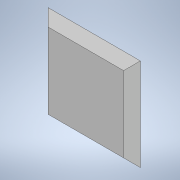
# Autodesk Inventor part: clear-square
Saved by Autodesk Inventor 2021 (Build 250183000, 183)
## iProperties
Created: 2020-12-08
Part Number: clear-square
Material: Generic
Document SubType Name: Modeling
Designer: Luke Kamols
Density: 1 g/cm^3
Appearance: Default
Author: Luke Kamols
Autodesk Inventor part; units mm, degrees
ref_plane "YZ Plane" through (0, 0, 0) normal (1, 0, 0) x (0, 1, 0)
ref_plane "XZ Plane" through (0, 0, 0) normal (0, 1, 0) x (-1, 0, 0)
ref_plane "XY Plane" through (0, 0, 0) normal (0, 0, 1) x (1, 0, 0)
sketch "Sketch1" plane through (0, 0, 0) normal (0, 0, 1) x (1, 0, 0)
  line L0 (0, 0) -> (44, 0)
  line L1 (44, 0) -> (44, 44)
  line L2 (44, 44) -> (0, 44)
  line L3 (0, 44) -> (0, 0)
  dimension "d0" = 44
  dimension "d1" = 44
  constraints: 8 end point, 2 parallel, 1 horizontal, 1 perpendicular
  measures "d0" distance of L2.end L1.end
  measures "d1" distance of L1.end L0.end
extrude "Extrusion1" add sketch "Sketch1" along normal blind 4
chamfer "Chamfer1" distance 4 angle 45 4 edges at (22, 44, 4) (44, 22, 4) (22, 0, 4) (0, 22, 4)
body "Solid1"
